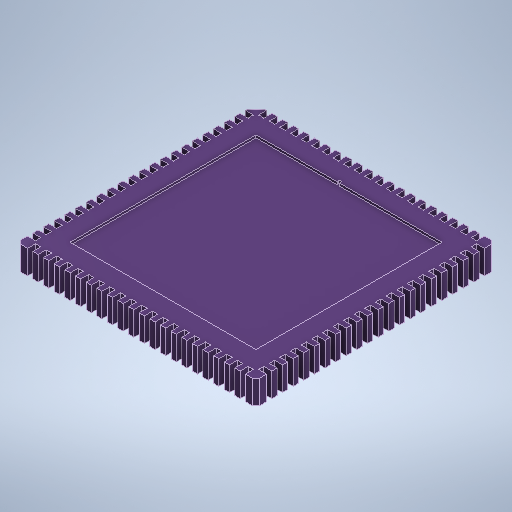
# Autodesk Inventor part: chip_body
Saved by Autodesk Inventor 2025 (Build 290162000, 162)
## iProperties
Created: 2025-09-08
Part Number: chip_body
Material: Purple ceramic
Document SubType Name: Modeling
Designer: jirne
Density: 1 g/cm^3
Appearance: Generic
Author: jirne
Autodesk Inventor part; units mm, degrees
ref_plane "YZ Plane" through (0, 0, 0) normal (1, 0, 0) x (0, 1, 0)
ref_plane "XZ Plane" through (0, 0, 0) normal (0, 1, 0) x (-1, 0, 0)
ref_plane "XY Plane" through (0, 0, 0) normal (0, 0, 1) x (1, 0, 0)
sketch "Sketch4" plane through (0, 0, 0) normal (0, 0, 1) x (1, 0, 0)
  line L0 (0, 0) -> (22.86, 0)
  line L1 (22.86, 0) -> (22.86, 22.86)
  line L2 (22.86, 22.86) -> (0, 22.86)
  line L3 (0, 22.86) -> (0, 0)
  dimension "d15" = 22.86
  constraints: 8 end point, 2 parallel, 2 perpendicular, 1 horizontal
  measures "d15" distance of L2.end L0.start
extrude "Extrusion2" add sketch "Sketch4" along normal blind 2.286
chamfer "Chamfer1" distance 0.8128 angle 45 1 edges at (0, 22.86, 1.143)
chamfer "Chamfer2" distance 0.3556 angle 45 3 edges at (22.86, 22.86, 1.143) (22.86, 0, 1.143) (0, 0, 1.143)
sketch "Sketch5" plane through (0, 0, 2.286) normal (0, 0, 1) x (1, 0, 0)
  line L0 (2.54, 2.54) -> (20.32, 2.54)
  line L1 (20.32, 2.54) -> (20.32, 20.32)
  line L2 (20.32, 20.32) -> (2.54, 20.32)
  line L3 (2.54, 20.32) -> (2.54, 2.54)
  line L4 (0.3556, 0) -> (22.5044, 0) projected
  line L5 (0, 22.0472) -> (0, 0.3556) projected
  point P0 (0, 0)
  dimension "d24" = 17.78
  dimension "d25" = 2.54
  dimension "d26" = 2.54
  constraints: 8 end point, 2 parallel, 2 perpendicular, 1 horizontal
  measures "d24" distance of L2.end L0.start
  measures "d25" distance from line of L4 point (2.54, 2.54)
  measures "d26" distance from line of L5 point (2.54, 2.54)
extrude "Extrusion3" cut sketch "Sketch5" against normal blind 0.254
sketch "Sketch6" plane through (0, 0, 2.286) normal (0, 0, 1) x (1, 0, 0)
  line L0 (10.287, 20.574) -> (10.541, 20.574)
  line L1 (10.541, 20.574) -> (10.541, 20.32)
  line L2 (10.541, 20.32) -> (10.287, 20.32)
  line L3 (10.287, 20.32) -> (10.287, 20.574)
  line L4 (2.54, 20.32) -> (20.32, 20.32) projected
  line L5 (2.54, 2.54) -> (2.54, 20.32) projected
  point P0 (0, 0)
  dimension "d29" = 0.254
  dimension "d53" = 7.747
  constraints: 8 end point, 2 parallel, 2 perpendicular, 1 horizontal, 1 point on line
  measures "d29" distance of L0.start L0.end
  measures "d53" distance between parallel lines of L3 L5
extrude "Extrusion4" cut sketch "Sketch6" against normal blind 0.254
sketch "Sketch7" plane through (0.3556, 0, 0) normal (0, -1, 0) x (1, 0, 0)
  line L0 (0, 0) -> (22.1488, 0) projected
  line L1 (0, 2.286) -> (22.1488, 2.286) projected
  line L2 (0.6604, 0) -> (1.1684, 0)
  line L3 (1.1684, 0) -> (1.1684, 2.286)
  line L4 (1.1684, 2.286) -> (0.6604, 2.286)
  line L5 (0.6604, 2.286) -> (0.6604, 0)
  point P0 (-0.3556, 0)
  dimension "d33" = 0.508
  dimension "d34" = 1.016
  constraints: 8 end point, 2 parallel, 2 point on line, 1 horizontal, 1 perpendicular
  measures "d33" distance between parallel lines of L3 L5
  measures "d34" distance of point (-0.356, 0) L2.start
extrude "Extrusion5" cut sketch "Sketch7" against normal blind 0.762
pattern_linear "Rectangular Pattern1" count 21 spacing 1.016 along (1, 0, 0) count 2 spacing 22.098 along (0, 1, 0) of "Extrusion5"
sketch "Sketch8" plane through (0, 22.0472, 0) normal (-1, 0, 0) x (0, 0, 1)
  line L0 (0, 0) -> (0, -21.6916) projected
  line L1 (2.286, 0) -> (2.286, -21.6916) projected
  line L2 (0, -0.2032) -> (2.286, -0.2032)
  line L3 (2.286, -0.2032) -> (2.286, -0.7112)
  line L4 (2.286, -0.7112) -> (0, -0.7112)
  line L5 (0, -0.7112) -> (0, -0.2032)
  line L6 (2.286, 0.8128) -> (0, 0.8128) projected
  point P0 (0, -22.0472)
  point P1 (0, -0.7112)
  point P2 (2.286, -0.2032)
  dimension "d43" = 0.508
  dimension "d44" = 1.016
  constraints: 8 end point, 2 parallel, 2 point on line, 1 horizontal, 1 perpendicular
  measures "d43" distance between parallel lines of L4 L2
  measures "d44" distance between parallel lines of L6 L2
extrude "Extrusion6" cut sketch "Sketch8" against normal blind 0.762
pattern_linear "Rectangular Pattern2" count 21 spacing 1.016 along (0, -1, 0) count 2 spacing 22.098 along (1, 0, 0) of "Extrusion6"
fillet "Fillet1" radius 0.127 2 edges at (10.287, 20.574, 2.159) (10.541, 20.574, 2.159)
body "Solid2"
